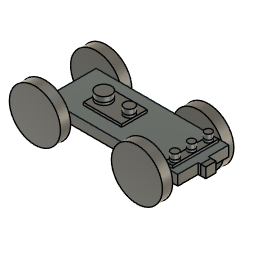
1100810 123 v2 (Autodesk Fusion 360 design; units mm, degrees)
Autodesk Fusion 360 part; units mm, degrees
note: some values were not read from the file. Set by a fixed rule: which sketch regions a step uses.
sketch "草图1" plane through (0, 0, 0) normal (0, 0, 1) x (1, 0, 0)
  line L0 (50, 100) -> (-50, 100)
  line L1 (-50, 100) -> (-50, -90)
  line L2 (-50, -90) -> (50, -90)
  line L3 (50, -90) -> (50, 100)
  constraint horizontal L0
  constraint vertical L1
  constraint horizontal L2
  constraint vertical L3
sketch "草图2" plane through (0, 0, 0) normal (0, 0, 1) x (1, 0, 0)
  line L0 (-100, 50) -> (100, 50)
  line L1 (100, 50) -> (100, -50)
  line L2 (100, -50) -> (-100, -50)
  line L3 (-100, -50) -> (-100, 50)
  constraint horizontal L0
  constraint vertical L1
  constraint horizontal L2
  constraint vertical L3
sketch "草图3" plane through (0, -50, 0) normal (0, -1, 0) x (1, 0, 0)
  line L0 (-100, 0) -> (100, 0)
  line L1 (100, 0) -> (100, 20)
  line L2 (100, 20) -> (-100, 20)
  line L3 (-100, 20) -> (-100, 0)
  circle A0 centre (-70, 0) radius 30
  circle A1 centre (70, 0) radius 30
  constraint coincident L0 A0.centre
  constraint tangent L3 A0
  constraint coincident L0 A1.centre
  constraint coincident L0.end A1
sketch "草图4" plane through (0, 50, 0) normal (0, 1, 0) x (-1, 0, 0)
  line L0 (-100, 0) -> (100, 0)
  line L1 (100, 0) -> (100, 20)
  line L2 (100, 20) -> (-100, 20)
  line L3 (-100, 20) -> (-100, 0)
  circle A0 centre (-70, 0) radius 30
  circle A1 centre (70, 0) radius 30
  constraint coincident L0 A0.centre
  constraint coincident L0 A1.centre
  constraint coincident L0.end A1
sketch "草图5" plane through (100, 0, 0) normal (1, 0, 0) x (0, 1, 0)
  line L0 (-50, 30) -> (50, 30)
  line L1 (50, 30) -> (50, 50)
  line L2 (50, 50) -> (-50, 50)
  line L3 (-50, 50) -> (-50, 30)
  line L4 (-50, 50) -> (50, 50)
  line L5 (50, 50) -> (50, 30)
  line L6 (50, 30) -> (-50, 30)
  line L7 (-50, 30) -> (-50, 50)
  constraint horizontal L4
  constraint vertical L5
  constraint horizontal L6
  constraint vertical L7
  constraint coincident L0.end L1.start
  constraint coincident L2.end L3.start
sketch "草图6" plane through (0, 0, 0) normal (0, 0, 1) x (1, 0, 0)
  line L0 (100, 50) -> (-100, 50)
  line L1 (-100, 50) -> (-100, -50)
  line L2 (-100, -50) -> (100, -50)
  line L3 (100, -50) -> (100, 50)
  constraint horizontal L0
  constraint vertical L1
  constraint horizontal L2
  constraint vertical L3
extrude "拉伸3" add sketch "草图6" along normal blind 20 makes body 1
sketch "草图7" plane through (0, -50, 0) normal (0, -1, 0) x (1, 0, 0)
  line L0 (-100, 0) -> (100, 0)
  line L1 (100, 0) -> (100, 20)
  line L2 (100, 20) -> (-100, 20)
  line L3 (-100, 20) -> (-100, 0)
  circle A0 centre (-100, 0) radius 50
  constraint coincident L0.start L3.end
extrude "拉伸4" add sketch "草图7" along normal blind 20 separate body contours L0 L2 L3 A0 | L0 L2 L3 A0 makes body 2
sketch "草图8" plane through (0, -50, 0) normal (0, -1, 0) x (1, 0, 0)
  line L0 (-100, 0) -> (100, 0)
  line L1 (100, 0) -> (100, 20)
  line L2 (100, 20) -> (-100, 20)
  line L3 (-100, 20) -> (-100, 0)
  circle A0 centre (100, 0) radius 50
  constraint coincident L0.end L1.start
extrude "拉伸5" add sketch "草图8" along normal blind 20 separate body contours L0 L1 L2 A0 | L0 L1 L2 A0 makes body 3
sketch "草图9" plane through (0, 50, 0) normal (0, 1, 0) x (-1, 0, 0)
  line L0 (-100, 0) -> (100, 0)
  line L1 (100, 0) -> (100, 20)
  line L2 (100, 20) -> (-100, 20)
  line L3 (-100, 20) -> (-100, 0)
  circle A0 centre (-100, 0) radius 50
  constraint coincident L0.start L3.end
extrude "拉伸6" add sketch "草图9" along normal blind 20 separate body contours L0 L2 L3 A0 | L0 L2 L3 A0 makes body 4
sketch "草图10" plane through (0, 50, 0) normal (0, 1, 0) x (-1, 0, 0)
  line L0 (-100, 0) -> (100, 0)
  line L1 (100, 0) -> (100, 20)
  line L2 (100, 20) -> (-100, 20)
  line L3 (-100, 20) -> (-100, 0)
  circle A0 centre (100, 0) radius 50
  constraint coincident L0.end L1.start
extrude "拉伸7" add sketch "草图10" along normal blind 20 separate body contours L0 L1 L2 A0 | L0 L1 L2 A0 makes body 5
move_body "移动4" bodies 1 2 5 3 4 to x (1, 0, 0) y (0, 1, 0) z (0, 0, 1) at (0, 0, 50)
sketch "草图11" plane through (100, 0, 0) normal (1, 0, 0) x (0, 1, 0)
  line L0 (-50, 50) -> (50, 50)
  line L1 (50, 50) -> (50, 70)
  line L2 (50, 70) -> (-50, 70)
  line L3 (-50, 70) -> (-50, 50)
  line L4 (-50, 70) -> (50, 70)
  line L5 (50, 70) -> (50, 50)
  line L6 (50, 50) -> (-50, 50)
  line L7 (-50, 50) -> (-50, 70)
  constraint horizontal L4
  constraint vertical L5
  constraint horizontal L6
  constraint vertical L7
  constraint coincident L0.end L1.start
  constraint coincident L2.end L3.start
extrude "拉伸8" add sketch "草图11" along normal blind 60 bodies 1 3 4
sketch "草图12" plane through (160, 0, 0) normal (1, 0, 0) x (0, 1, 0)
  line L0 (-50, 50) -> (50, 50)
  line L1 (50, 50) -> (50, 70)
  line L2 (50, 70) -> (-50, 70)
  line L3 (-50, 70) -> (-50, 50)
  line L4 (-10, 70) -> (10, 70)
  line L5 (10, 70) -> (10, 50)
  line L6 (10, 50) -> (-10, 50)
  line L7 (-10, 50) -> (-10, 70)
  constraint horizontal L4
  constraint vertical L5
  constraint horizontal L6
  constraint vertical L7
  constraint coincident L0 L5.end
  constraint coincident L2 L4.start
extrude "拉伸9" add sketch "草图12" along normal blind 5 contours L0 L2 L4 L5 L6 L7 bodies 1
sketch "草图13" plane through (165, 0, 0) normal (1, 0, 0) x (0, 1, 0)
  line L0 (-10, 50) -> (10, 50)
  line L1 (10, 50) -> (10, 70)
  line L2 (10, 70) -> (-10, 70)
  line L3 (-10, 70) -> (-10, 50)
  line L4 (-10, 70) -> (10, 70)
  line L5 (10, 70) -> (10, 50)
  line L6 (10, 50) -> (-10, 50)
  line L7 (-10, 50) -> (-10, 70)
  constraint horizontal L4
  constraint vertical L5
  constraint horizontal L6
  constraint vertical L7
  constraint coincident L0.end L1.start
  constraint coincident L2.end L3.start
extrude "拉伸10" add sketch "草图13" along normal blind 10 separate body makes body 6
sketch "草图14" plane through (0, 0, 70) normal (0, 0, 1) x (-1, 0, 0)
  line L0 (-145.8258, -50) -> (-54.1742, -50)
  line L1 (-54.1742, -50) -> (100, -50)
  line L2 (100, -50) -> (100, 50)
  line L3 (100, 50) -> (-54.1742, 50)
  line L4 (-54.1742, 50) -> (-145.8258, 50)
  line L5 (-145.8258, 50) -> (-160, 50)
  line L6 (-160, 50) -> (-160, 10)
  line L7 (-160, 10) -> (-165, 10)
  line L8 (-165, 10) -> (-165, -10)
  line L9 (-165, -10) -> (-160, -10)
  line L10 (-160, -10) -> (-160, -50)
  line L11 (-160, -50) -> (-145.8258, -50)
  line L12 (-145, 45) -> (-130, 45)
  line L13 (-130, 45) -> (-130, -45)
  line L14 (-130, -45) -> (-145, -45)
  line L15 (-145, -45) -> (-145, 45)
  constraint horizontal L12
  constraint vertical L13
  constraint horizontal L14
  constraint vertical L15
extrude "拉伸11" add sketch "草图14" along normal blind 5 contours L12 L13 L14 L15 bodies 1
sketch "草图15" plane through (0, 0, 70) normal (0, 0, 1) x (-1, 0, 0)
  line L0 (-145, -45) -> (-145, 45)
  line L1 (-145, 45) -> (-130, 45)
  line L2 (-130, 45) -> (-130, -45)
  line L3 (-130, -45) -> (-145, -45)
  line L4 (-145.8258, -50) -> (-54.1742, -50)
  line L5 (-54.1742, -50) -> (100, -50)
  line L6 (100, -50) -> (100, 50)
  line L7 (100, 50) -> (-54.1742, 50)
  line L8 (-54.1742, 50) -> (-145.8258, 50)
  line L9 (-145.8258, 50) -> (-160, 50)
  line L10 (-160, 50) -> (-160, 10)
  line L11 (-160, 10) -> (-165, 10)
  line L12 (-165, 10) -> (-165, -10)
  line L13 (-165, -10) -> (-160, -10)
  line L14 (-160, -10) -> (-160, -50)
  line L15 (-160, -50) -> (-145.8258, -50)
sketch "草图16" plane through (0, 0, 75) normal (0, 0, 1) x (-1, 0, 0)
  line L0 (-145, -45) -> (-130, -45)
  line L1 (-130, -45) -> (-130, 45)
  line L2 (-130, 45) -> (-145, 45)
  line L3 (-145, 45) -> (-145, -45)
  circle A0 centre (-137.5, 33.0439) radius 7.5
  constraint tangent L1 A0
extrude "拉伸12" add sketch "草图16" along normal blind 5 contours A0 bodies 1
sketch "草图17" plane through (0, 0, 0) normal (0, 1, 0) x (1, 0, 0)
extrude "拉伸13" add 1 faces at (137.0539, -34.9985, 80) along direction (0, 0, 1) blind 10 separate body on bodies 1 makes body 7
sketch "草图18" plane through (0, 0, 75) normal (0, 0, 1) x (-1, 0, 0)
  arc A0 (-145, 33.0439) -> (-130, 33.0439) centre (-137.5, 33.0439) ccw
  line L0 (-145, 33.0439) -> (-145, -45)
  line L1 (-145, -45) -> (-130, -45)
  line L2 (-130, -45) -> (-130, 33.0439)
  circle A1 centre (-137, 0) radius 7
  constraint tangent L2 A1
extrude "拉伸14" add sketch "草图18" along normal blind 5 contours A1 bodies 1
extrude "拉伸15" add 1 faces at (136.1475, 2.172, 80) along direction (0, 0, 1) blind 10 separate body on bodies 1 makes body 8
sketch "草图19" plane through (0, 0, 75) normal (0, 0, 1) x (-1, 0, 0)
  arc A0 (-145, 33.0439) -> (-130, 33.0439) centre (-137.5, 33.0439) ccw
  line L0 (-145, 33.0439) -> (-145, -45)
  line L1 (-145, -45) -> (-130, -45)
  line L2 (-130, -45) -> (-130, 0)
  circle A1 centre (-137, 0) radius 7
  line L3 (-130, 0) -> (-130, 33.0439)
  circle A2 centre (-137, -33) radius 7
  constraint tangent L2 A2
extrude "拉伸16" add sketch "草图19" along normal blind 5 contours A2 bodies 1
extrude "拉伸17" add 1 faces at (137.5192, 32.646, 80) along direction (0, 0, 1) blind 10 separate body on bodies 1 makes body 9
sketch "草图20" plane through (0, 0, 70) normal (0, 0, 1) x (-1, 0, 0)
  line L0 (-25, 25) -> (50, 25)
  line L1 (50, 25) -> (50, -25)
  line L2 (50, -25) -> (-25, -25)
  line L3 (-25, -25) -> (-25, 25)
  constraint horizontal L0
  constraint vertical L1
  constraint horizontal L2
  constraint vertical L3
extrude "拉伸18" add sketch "草图20" along normal blind 5 bodies 1
sketch "草图21" plane through (0, 0, 75) normal (0, 0, 1) x (-1, 0, 0)
  line L0 (-25, -25) -> (50, -25)
  line L1 (50, -25) -> (50, 25)
  line L2 (50, 25) -> (-25, 25)
  line L3 (-25, 25) -> (-25, -25)
  circle A0 centre (-15, 0) radius 10
  constraint tangent L3 A0
extrude "拉伸19" add sketch "草图21" along normal blind 5 contours A0 bodies 1
extrude "拉伸20" add 1 faces at (12.9217, 2.6061, 80) along direction (0, 0, 1) blind 10 separate body on bodies 1 makes body 10
sketch "草图22" plane through (0, 0, 75) normal (0, 0, 1) x (-1, 0, 0)
  line L0 (-25, -25) -> (50, -25)
  line L1 (50, -25) -> (50, 25)
  line L2 (50, 25) -> (-25, 25)
  line L3 (-25, 25) -> (-25, 0)
  circle A0 centre (-15, 0) radius 10
  line L4 (-25, 0) -> (-25, -25)
  circle A1 centre (35, 0) radius 15
  constraint tangent L1 A1
extrude "拉伸21" add sketch "草图22" along normal blind 5 contours A1 bodies 1
extrude "拉伸22" add 1 faces at (-28.2948, 2.5011, 80) along direction (0, 0, 1) blind 10 separate body on bodies 1 makes body 11
copy_body "实体->零部件1" bodies 1 removing the originals makes body 12 in component "base_link"
copy_body "实体->零部件2" bodies 2 removing the originals makes body 13 in component "right_wheel"
copy_body "实体->零部件3" bodies 5 removing the originals makes body 14 in component "left_wheel"
copy_body "实体->零部件4" bodies 6 removing the originals makes body 15 in component "Bumper"
copy_body "实体->零部件5" bodies 7 removing the originals makes body 16 in component "Lidar"
copy_body "实体->零部件6" bodies 8 removing the originals makes body 17 in component "Depth_Camera"
copy_body "实体->零部件7" bodies 9 removing the originals makes body 18 in component "Camera"
copy_body "实体->零部件8" bodies 10 removing the originals makes body 19 in component "IMU"
copy_body "实体->零部件9" bodies 11 removing the originals makes body 20 in component "GPS"
component "base_link" placed x (1, 0, 0) y (0, 1, 0) z (0, 0, 1) at (0, 0, 0)
component "right_wheel" placed x (1, 0, 0) y (0, 1, 0) z (0, 0, 1) at (0, 0, 0)
component "left_wheel" placed x (1, 0, 0) y (0, 1, 0) z (0, 0, 1) at (0, 0, 0)
component "Bumper" placed x (1, 0, 0) y (0, 1, 0) z (0, 0, 1) at (0, 0, 0)
component "Lidar" placed x (1, 0, 0) y (0, 1, 0) z (0, 0, 1) at (0, 0, 0)
component "Depth_Camera" placed x (1, 0, 0) y (0, 1, 0) z (0, 0, 1) at (0, 0, 0)
component "Camera" placed x (1, 0, 0) y (0, 1, 0) z (0, 0, 1) at (0, 0, 0)
component "IMU" placed x (1, 0, 0) y (0, 1, 0) z (0, 0, 1) at (0, 0, 0)
component "GPS" placed x (1, 0, 0) y (0, 1, 0) z (0, 0, 1) at (0, 0, 0)
named bodies: "base_link", "right_wheel", "left_wheel", "Bumper", "Lidar", "Depth_Camera", "Camera", "IMU", "GPS"
